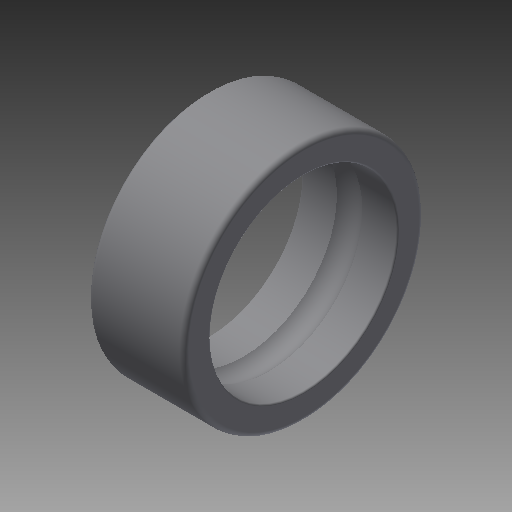
# Autodesk Inventor part: W 618/2 X_PART2
Saved by Autodesk Inventor 2018.3 (Build 223284000, 284)
## iProperties
Category: PARTsolutions
Company: SKF
Created: 2018-08-18
Part Number: W 618/2 X_PART2
Material: Generic
Catalog Web Link: www.cadenas.de
Description: -Deep groove ball bearings
Vendor: SKF
Document SubType Name: Modeling
Designer: psadmin
Manufacturer: SKF
Mass: 0.0148519 g
Surface Area: 0.704324 cm^2
Volume: 0.0148519 cm^3
Density: 1 g/cm^3
Appearance: PSOLRGB-175-175-175
PSOL_IDENT_0: {$CADENAS_DATA\23d-libs\skf\bearings_units_and_housings\ball_bearings\deep_groove_ball_bearings\bb1_
PSOL_IDENT_1: 001_101.prj},197 {VTYP=3D},{NB=W 618/2 X_PART2},{LINA=W 618/2 X_PART2},{NN=BB1_001_101_PART2},{NOPRJ=
PSOL_IDENT_2: TRUE},{DATE=18.08.2018 08:27:38},{GEOMDATE=08.08.2018 12:16:40},{VERSION=},{LINEID=18450},{WBVAR=},{
PSOL_IDENT_3: WBNUMERIC=}  {NB=W 618/2 X_PART2},{LINA=W 618/2 X_PART2},{KT=DUMMY},{PRODUCTID=},{DESIGNATION=W 618/
PSOL_IDENT_4: 2 X},{DD=2.00},{D=5.000},{B=2.000},{C=0.000},{DD1=2.70},{DD2=0.0},{D1=3.90},{D2=0.00},{D3=0.00},{D4=
PSOL_IDENT_5: 0.000},{HH=MIN},{BB=0.000},{FF=0.00},{R0MAX=MIN},{R0=MIN},{R12=0.10},{PITCH=3.30},{DW=0.800},{DDAMIN=
PSOL_IDENT_6: 2.600},{DDAMAX=MIN},{DDBMIN=MIN},{DDBMAX=MIN},{DBMIN=MIN},{DAMAX=4.200},{BBAMIN=MIN},{CAMAX=MIN},{RA
PSOL_IDENT_7: MAX=0.100},{LOAD1=0.094},{LOAD2=0.025},{LOAD3=0.001},{SPEED1=200000},{SPEED2=120000},{KR=0.020},{F0=
PSOL_IDENT_8: 6.500},{Z=6},{II=1},{MASS=0.000},{BEARING=W 618/2 X},{RING=},{HELP=0.550},{HELP2=0.550},{DD1ALG=1.35
PSOL_IDENT_9: 0},{YALG=1.350},{PITCH1=3.300},{DW1=0.800},{YALG1=1.950},{HALG1=0.550},{SH=1.350},{CU=0.240},{DESIGN=
PSOL_IDENT_10: dgbbw},{HALG=0.35},{B1=0},{ALGO=1.000}
NT: Deep groove ball bearings
NB: W 618/2 X_PART2
NBSYN: $DESIGNATION._PART2
LINA: W 618/2 X_PART2
SUPPLIER: SKF
ARTICLENO: W 618/2 X_PART2
BOMINFO: W 618/2 X_PART2
CREATOR: CADENAS GmbH
Title: W 618/2 X_PART2
Author: Cadenas PARTsolutions
Comments: Deep groove ball bearings
Autodesk Inventor part; units mm, degrees
ref_plane "YZ Plane" through (0, 0, 0) normal (1, 0, 0) x (0, 1, 0)
ref_plane "XZ Plane" through (0, 0, 0) normal (0, 1, 0) x (-1, 0, 0)
ref_plane "XY Plane" through (0, 0, 0) normal (0, 0, 1) x (1, 0, 0)
sketch "Sketch_7" plane through (0, 0, 0) normal (0, 0, 1) x (1, 0, 0)
  line L0 (2, 0) -> (-2, 0)
  arc A0 (0, 1.9833) -> (0.0333, 1.95) centre (0.0333, 1.9833) ccw
  line L1 (0.0333, 1.95) -> (0.7354, 1.95)
  arc A1 (1.2646, 1.95) -> (0.7354, 1.95) centre (1, 1.65) ccw
  line L2 (1.2646, 1.95) -> (1.9667, 1.95)
  arc A2 (1.9667, 1.95) -> (2, 1.9833) centre (1.9667, 1.9833) ccw
  line L3 (2, 1.9833) -> (2, 2.4)
  arc A3 (2, 2.4) -> (1.9, 2.5) centre (1.9, 2.4) ccw
  line L4 (1.9, 2.5) -> (0.1, 2.5)
  arc A4 (0.1, 2.5) -> (0, 2.4) centre (0.1, 2.4) ccw
  line L5 (0, 2.4) -> (0, 1.9833)
  constraints: 12 end point, 10 point on circle, 5 centre point
revolve "Revolution1" add sketch "Sketch_7" angle 360 about axis through (2, 0, 0) along (1, 0, 0)
body "Solid1"
